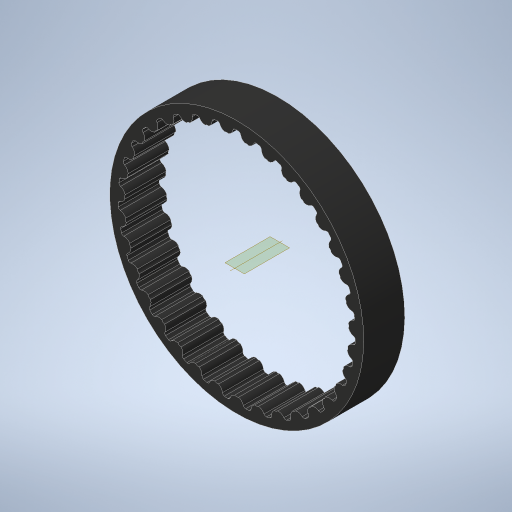
# Autodesk Inventor part: belt tooth
Saved by Autodesk Inventor 2023.3 (Build 273359000, 359)
## iProperties
Created: 2024-02-03
Part Number: belt tooth
Material: Rubber, Silicone
Document SubType Name: Modeling
Designer: mavericks
Density: 1.25 g/cm^3
Appearance: Rubber - Black
Author: mavericks
Autodesk Inventor part; units mm, degrees
(part 1 of 2)
ref_plane "YZ Plane" through (0, 0, 0) normal (1, 0, 0) x (0, 1, 0)
ref_plane "XZ Plane" through (0, 0, 0) normal (0, 1, 0) x (-1, 0, 0)
ref_plane "XY Plane" through (0, 0, 0) normal (0, 0, 1) x (1, 0, 0)
sketch "Sketch1" plane through (0, 0, 0) normal (0, 0, 1) x (1, 0, 0)
  line L0 (3.873, 1.9) -> (5, 1.9) construction
  arc A0 (3.3889, 2.275) -> (3.873, 1.9) centre (3.873, 2.4) ccw
  arc A1 (3.3889, 2.275) -> (2.3532, 3.341) centre (1.9365, 1.9) ccw
  arc A2 (1.5198, 3.341) -> (2.3532, 3.341) centre (1.9365, 4.0627) ccw
  arc A3 (1.5198, 3.341) -> (0.4841, 2.275) centre (1.9365, 1.9) ccw
  arc A4 (0, 1.9) -> (0.4841, 2.275) centre (0, 2.4) ccw
  line L1 (0, 0) -> (6.35, 0) construction
  line L2 (0, 1.9) -> (0, 0)
  line L3 (3.873, 1.9) -> (3.873, 0)
  line L4 (3.873, 0) -> (0, 0)
  dimension "d1" = 1.127
  dimension "d2" = 0.5
  dimension "d3" = 1.5
  dimension "d4" = 0.8333
  dimension "d5" = 1.5
  dimension "d6" = 0.5
  dimension "d7" = 1.9
  dimension "d8" = 2.4
  dimension "d9" = 1.9365
  dimension "d10" = 1.9365
  dimension "d11" = 1.6626
  dimension "d12" = 0.5
  dimension "d13" = 1.9
  dimension "d14" = 0
  dimension "d15" = 6.35
  dimension "d16" = 0.4841
  dimension "d17" = 1.0357
  dimension "d18" = 0.375
  dimension "d19" = 1.066
  constraints: 10 end point, 10 point on circle, 5 centre point, 2 perpendicular, 1 coincident, 1 horizontal, 1 point on line
  measures "d1" distance of L0.start L0.end
  measures "d2" radius of A0
  measures "d3" radius of A1
  measures "d4" radius of A2
  measures "d5" radius of A3
  measures "d6" radius of A4
  measures "d7" distance between parallel lines of L1 L0
  measures "d8" distance from line of L1 A4.centre
  measures "d9" horizontal distance of A2.centre A4.centre
  measures "d10" horizontal distance of A0.centre A2.centre
  measures "d11" vertical distance of A2.centre A0.centre
  measures "d12" vertical distance of A1.centre A0.centre
  measures "d13" distance from line of L1 A1.centre
  measures "d14" horizontal distance of L1.start A4.centre
  measures "d15" distance of L1.start L1.end
  measures "d16" horizontal distance of L0.start A0.start
  measures "d17" horizontal distance of A3.end A3.start
  measures "d18" vertical distance of L2.start A3.end
  measures "d19" vertical distance of A3.end A3.start
extrude "Extrusion1" add sketch "Sketch1" along normal mid plane 9
ref_plane "Work Plane1" through (0, 27.8521, 4.5) normal (0, -1, 0) x (1, 0, 0)
sketch "Sketch2" plane through (0, 27.8521, 4.5) normal (0, -1, 0) x (1, 0, 0)
  line L0 (1.5198, -9) -> (1.5198, 0) construction
  line L1 (2.3532, 0) -> (2.3532, 0) construction
  line L2 (2.3532, 0) -> (2.3532, -9) construction
  line L3 (1.5198, -9) -> (2.3532, -9) construction
  line L4 (3.873, -9) -> (0, -9) construction
  line L5 (1.9365, -9) -> (1.9365, 0)
  line L6 (2.3532, 0) -> (2.3532, 0) construction
  point P0 (0, -4.5)
  constraints: 2 end point, 1 midpoint, 1 point on line
pattern_circular "Circular Pattern1" count 35 over 360 about axis through (1.9365, 27.8521, -4.5) along (0, 0, 1) of "Extrusion1"
sketch "Sketch3" plane through (0, 0, 4.5) normal (0, 0, 1) x (1, 0, 0)
  arc A0 (3.3889, 2.275) -> (2.3532, 3.341) centre (1.9365, 1.9) ccw construction
  arc A1 (3.3889, 2.275) -> (3.873, 1.9) centre (3.873, 2.4) ccw construction
  line L0 (3.873, 1.9) -> (3.873, 0) construction
  line L1 (3.873, 0) -> (0, 0) construction
  line L2 (0, 0) -> (0, 1.9) construction
  arc A2 (0, 1.9) -> (0.4841, 2.275) centre (0, 2.4) ccw construction
  arc A3 (1.5198, 3.341) -> (0.4841, 2.275) centre (1.9365, 1.9) ccw construction
  arc A4 (1.5198, 3.341) -> (2.3532, 3.341) centre (1.9365, 4.0627) ccw construction
  arc A5 (7.9325, 2.9454) -> (6.7231, 3.8093) centre (6.5704, 2.3171) ccw construction
  arc A6 (7.9325, 2.9454) -> (8.4758, 2.6628) centre (8.3865, 3.1548) ccw construction
  line L3 (8.4758, 2.6628) -> (8.815, 0.7934) construction
  line L4 (8.815, 0.7934) -> (5.0043, 0.1018) construction
  line L5 (5.0043, 0.1018) -> (4.665, 1.9713) construction
  arc A7 (4.665, 1.9713) -> (5.0744, 2.4267) centre (4.5758, 2.4633) ccw construction
  arc A8 (5.9032, 3.6605) -> (5.0744, 2.4267) centre (6.5704, 2.3171) ccw construction
  arc A9 (5.9032, 3.6605) -> (6.7231, 3.8093) centre (6.1843, 4.445) ccw construction
  arc A10 (12.2834, 4.4163) -> (10.9392, 5.0503) centre (11.0554, 3.5548) ccw construction
  arc A11 (12.2834, 4.4163) -> (12.8684, 4.2353) centre (12.6927, 4.7034) ccw construction
  line L6 (12.8684, 4.2353) -> (13.536, 2.4564) construction
  line L7 (13.536, 2.4564) -> (9.91, 1.0956) construction
  line L8 (9.91, 1.0956) -> (9.2424, 2.8744) construction
  arc A12 (9.2424, 2.8744) -> (9.5639, 3.3956) centre (9.0667, 3.3425) ccw construction
  arc A13 (10.159, 4.7575) -> (9.5639, 3.3956) centre (11.0554, 3.5548) ccw construction
  arc A14 (10.159, 4.7575) -> (10.9392, 5.0503) centre (10.2955, 5.5796) ccw construction
  arc A15 (16.3018, 6.6404) -> (14.8659, 7.0243) centre (15.2473, 5.5736) ccw construction
  arc A16 (16.3018, 6.6404) -> (16.9097, 6.5668) centre (16.6532, 6.996) ccw construction
  line L9 (16.9097, 6.5668) -> (17.8842, 4.9357) construction
  line L10 (17.8842, 4.9357) -> (14.5594, 2.9493) construction
  line L11 (14.5594, 2.9493) -> (13.5849, 4.5803) construction
  arc A17 (13.5849, 4.5803) -> (13.8082, 5.1506) centre (13.3285, 5.0096) ccw construction
  arc A18 (14.1506, 6.5968) -> (13.8082, 5.1506) centre (15.2473, 5.5736) ccw construction
  arc A19 (14.1506, 6.5968) -> (14.8659, 7.0243) centre (14.1381, 7.4301) ccw construction
  arc A20 (19.8584, 9.5463) -> (18.3771, 9.6676) centre (19.0114, 8.3083) ccw construction
  arc A21 (19.8584, 9.5463) -> (20.4697, 9.5824) centre (20.1407, 9.9589) ccw construction
  line L12 (20.4697, 9.5824) -> (21.7198, 8.1516) construction
  line L13 (21.7198, 8.1516) -> (18.8032, 5.6034) construction
  line L14 (18.8032, 5.6034) -> (17.5531, 7.0342) construction
  arc A22 (17.5531, 7.0342) -> (17.6709, 7.6351) centre (17.2241, 7.4108) ccw construction
  arc A23 (17.7495, 9.1193) -> (17.6709, 7.6351) centre (19.0114, 8.3083) ccw construction
  arc A24 (17.7495, 9.1193) -> (18.3771, 9.6676) centre (17.5885, 9.937) ccw construction
  arc A25 (22.839, 13.0406) -> (21.3599, 12.8954) centre (22.2267, 11.6712) ccw construction
  arc A26 (22.839, 13.0406) -> (23.4341, 13.1852) centre (23.0431, 13.497) ccw construction
  line L15 (23.4341, 13.1852) -> (24.9195, 12.0006) construction
  line L16 (24.9195, 12.0006) -> (22.5048, 8.9726) construction
  line L17 (22.5048, 8.9726) -> (21.0193, 10.1572) construction
  arc A27 (21.0193, 10.1572) -> (21.0279, 10.7695) centre (20.6284, 10.469) ccw construction
  arc A28 (20.8403, 12.2439) -> (21.0279, 10.7695) centre (22.2267, 11.6712) ccw construction
  arc A29 (20.8403, 12.2439) -> (21.3599, 12.8954) centre (20.5358, 13.0196) ccw construction
  arc A30 (25.1478, 17.0109) -> (23.7183, 16.604) centre (24.7898, 15.5542) ccw construction
  arc A31 (25.1478, 17.0109) -> (25.7075, 17.2595) centre (25.2672, 17.4964) ccw construction
  line L18 (25.7075, 17.2595) -> (27.3806, 16.3591) construction
  line L19 (27.3806, 16.3591) -> (25.5453, 12.9486) construction
  line L20 (25.5453, 12.9486) -> (23.8722, 13.849) construction
  arc A32 (23.8722, 13.849) -> (23.7714, 14.453) centre (23.4319, 14.0859) ccw construction
  arc A33 (23.3235, 15.8701) -> (23.7714, 14.453) centre (24.7898, 15.5542) ccw construction
  arc A34 (23.3235, 15.8701) -> (23.7183, 16.604) centre (22.8854, 16.579) ccw construction
  arc A35 (26.7106, 21.3296) -> (25.3767, 20.674) centre (26.6184, 19.8325) ccw construction
  arc A36 (26.7106, 21.3296) -> (27.2168, 21.6742) centre (26.7413, 21.8287) ccw construction
  line L21 (27.2168, 21.6742) -> (29.0238, 21.0871) construction
  line L22 (29.0238, 21.0871) -> (27.827, 17.4036) construction
  line L23 (27.827, 17.4036) -> (26.02, 17.9908) construction
  arc A37 (26.02, 17.9908) -> (25.813, 18.5671) centre (25.5445, 18.1453) ccw construction
  arc A38 (25.1192, 19.8815) -> (25.813, 18.5671) centre (26.6184, 19.8325) ccw construction
  arc A39 (25.1192, 19.8815) -> (25.3767, 20.674) centre (24.5616, 20.5008) ccw construction
  arc A40 (27.4771, 25.858) -> (26.2817, 24.9748) centre (27.6537, 24.3685) ccw construction
  arc A41 (27.4771, 25.858) -> (27.9137, 26.2874) centre (27.4182, 26.3546) ccw construction
  line L24 (27.9137, 26.2874) -> (29.7965, 26.0324) construction
  line L25 (29.7965, 26.0324) -> (29.2766, 22.1945) construction
  line L26 (29.2766, 22.1945) -> (27.3938, 22.4495) construction
  arc A42 (27.3938, 22.4495) -> (27.0872, 22.9796) centre (26.8983, 22.5166) ccw construction
  arc A43 (26.1699, 24.149) -> (27.0872, 22.9796) centre (27.6537, 24.3685) ccw construction
  arc A44 (26.1699, 24.149) -> (26.2817, 24.9748) centre (25.5107, 24.6588) ccw construction
  arc A45 (27.4227, 30.4505) -> (26.4043, 29.3681) centre (27.8625, 29.0165) ccw construction
  arc A46 (27.4227, 30.4505) -> (27.7756, 30.951) centre (27.2761, 30.9286) ccw construction
  line L27 (27.7756, 30.951) -> (29.6737, 31.0362) construction
  line L28 (29.6737, 31.0362) -> (29.8474, 27.1672) construction
  line L29 (29.8474, 27.1672) -> (27.9494, 27.0819) construction
  arc A47 (27.9494, 27.0819) -> (27.553, 27.5487) centre (27.4499, 27.0595) ccw construction
  arc A48 (26.4417, 28.5356) -> (27.553, 27.5487) centre (27.8625, 29.0165) ccw construction
  arc A49 (26.4417, 28.5356) -> (26.4043, 29.3681) centre (25.702, 28.9194) ccw construction
  arc A50 (26.5492, 34.9595) -> (25.7404, 33.7126) centre (27.2379, 33.627) ccw construction
  arc A51 (26.5492, 34.9595) -> (26.807, 35.5149) centre (26.3196, 35.4037) ccw construction
  line L30 (26.807, 35.5149) -> (28.6594, 35.9377) construction
  line L31 (28.6594, 35.9377) -> (29.5212, 32.1619) construction
  line L32 (29.5212, 32.1619) -> (27.6688, 31.7391) construction
  arc A52 (27.6688, 31.7391) -> (27.1955, 32.1276) centre (27.1814, 31.6278) ccw construction
  arc A53 (25.9258, 32.9001) -> (27.1955, 32.1276) centre (27.2379, 33.627) ccw construction
  arc A54 (25.9258, 32.9001) -> (25.7404, 33.7126) centre (25.1295, 33.1458) ccw construction
  arc A55 (24.8845, 39.2401) -> (24.3114, 37.8687) centre (25.8002, 38.0519) ccw construction
  arc A56 (24.8845, 39.2401) -> (25.0391, 39.8326) centre (24.5793, 39.6361) ccw construction
  line L33 (25.0391, 39.8326) -> (26.7862, 40.5794) construction
  line L34 (26.7862, 40.5794) -> (28.3084, 37.018) construction
  line L35 (28.3084, 37.018) -> (26.5613, 36.2713) construction
  arc A57 (26.5613, 36.2713) -> (26.0262, 36.5691) centre (26.1015, 36.0748) ccw construction
  arc A58 (24.6389, 37.1025) -> (26.0262, 36.5691) centre (25.8002, 38.0519) ccw construction
  arc A59 (24.6389, 37.1025) -> (24.3114, 37.8687) centre (23.8116, 37.202) ccw construction
  arc A60 (22.4824, 43.1546) -> (22.1633, 41.703) centre (23.5954, 42.1491) ccw construction
  arc A61 (22.4824, 43.1546) -> (22.5286, 43.7652) centre (22.1113, 43.4898) ccw construction
  line L36 (22.5286, 43.7652) -> (24.1143, 44.8119) construction
  line L37 (24.1143, 44.8119) -> (26.2479, 41.5796) construction
  line L38 (26.2479, 41.5796) -> (24.6622, 40.5329) construction
  arc A62 (24.6622, 40.5329) -> (24.0826, 40.7304) centre (24.245, 40.2575) ccw construction
  arc A63 (22.6224, 41.0075) -> (24.0826, 40.7304) centre (23.5954, 42.1491) ccw construction
  arc A64 (22.6224, 41.0075) -> (22.1633, 41.703) centre (21.7905, 40.9577) ccw construction
  arc A65 (19.4198, 46.5773) -> (19.3651, 45.092) centre (20.6945, 45.7867) ccw construction
  arc A66 (19.4198, 46.5773) -> (19.3563, 47.1863) centre (18.9949, 46.8408) ccw construction
  line L39 (19.3563, 47.1863) -> (20.7296, 48.4994) construction
  line L40 (20.7296, 48.4994) -> (23.4061, 45.7) construction
  line L41 (23.4061, 45.7) -> (22.0328, 44.387) construction
  arc A67 (22.0328, 44.387) -> (21.4272, 44.4777) centre (21.6714, 44.0414) ccw construction
  arc A68 (19.941, 44.4897) -> (21.4272, 44.4777) centre (20.6945, 45.7867) ccw construction
  arc A69 (19.941, 44.4897) -> (19.3651, 45.092) centre (19.1314, 44.2921) ccw construction
  arc A70 (15.7954, 49.3981) -> (16.0067, 47.927) centre (17.1908, 48.8478) ccw construction
  arc A71 (15.7954, 49.3981) -> (15.6241, 49.9861) centre (15.3302, 49.5816) ccw construction
  line L42 (15.6241, 49.9861) -> (16.7409, 51.5232) construction
  line L43 (16.7409, 51.5232) -> (19.8742, 49.2467) construction
  line L44 (19.8742, 49.2467) -> (18.7574, 47.7096) construction
  arc A72 (18.7574, 47.7096) -> (18.1453, 47.6908) centre (18.4635, 47.3051) ccw construction
  arc A73 (16.6809, 47.4371) -> (18.1453, 47.6908) centre (17.1908, 48.8478) ccw construction
  arc A74 (16.6809, 47.4371) -> (16.0067, 47.927) centre (15.9196, 47.0982) ccw construction
  arc A75 (11.7254, 51.5265) -> (12.1961, 50.1167) centre (13.1967, 51.2342) ccw construction
  arc A76 (11.7254, 51.5265) -> (11.452, 52.0744) centre (11.235, 51.6239) ccw construction
  line L45 (11.452, 52.0744) -> (12.2764, 53.7862) construction
  line L46 (12.2764, 53.7862) -> (15.7658, 52.1058) construction
  line L47 (15.7658, 52.1058) -> (14.9414, 50.394) construction
  arc A77 (14.9414, 50.394) -> (14.3425, 50.2661) centre (14.7245, 49.9435) ccw construction
  arc A78 (12.9469, 49.7551) -> (14.3425, 50.2661) centre (13.1967, 51.2342) ccw construction
  arc A79 (12.9469, 49.7551) -> (12.1961, 50.1167) centre (12.2584, 49.2857) ccw construction
  arc A80 (7.3409, 52.8939) -> (8.0557, 51.5908) centre (8.8407, 52.869) ccw construction
  arc A81 (7.3409, 52.8939) -> (6.974, 53.3842) centre (6.841, 52.9022) ccw construction
  line L48 (6.974, 53.3842) -> (7.4795, 55.2157) construction
  line L49 (7.4795, 55.2157) -> (11.2129, 54.1853) construction
  line L50 (11.2129, 54.1853) -> (10.7074, 52.3538) construction
  arc A82 (10.7074, 52.3538) -> (10.141, 52.1211) centre (10.5744, 51.8718) ccw construction
  arc A83 (8.859, 51.3691) -> (10.141, 52.1211) centre (8.8407, 52.869) ccw construction
  arc A84 (8.859, 51.3691) -> (8.0557, 51.5908) centre (8.2654, 50.7843) ccw construction
  arc A85 (2.7827, 53.4565) -> (3.7187, 52.3019) centre (4.2628, 53.6998) ccw construction
  arc A86 (2.7827, 53.4565) -> (2.3341, 53.8733) centre (2.2893, 53.3754) ccw construction
  line L51 (2.3341, 53.8733) -> (2.5044, 55.7657) construction
  line L52 (2.5044, 55.7657) -> (6.3618, 55.4185) construction
  line L53 (6.3618, 55.4185) -> (6.1915, 53.5262) construction
  arc A87 (6.1915, 53.5262) -> (5.6757, 53.1961) centre (6.1467, 53.0282) ccw construction
  arc A88 (4.5486, 52.2272) -> (5.6757, 53.1961) centre (4.2628, 53.6998) ccw construction
  arc A89 (4.5486, 52.2272) -> (3.7187, 52.3019) centre (4.069, 51.5458) ccw construction
  arc A90 (-1.8027, 53.1961) -> (-0.6757, 52.2272) centre (-0.3898, 53.6998) ccw construction
  arc A91 (-1.8027, 53.1961) -> (-2.3185, 53.5262) centre (-2.2737, 53.0282) ccw construction
  line L54 (-2.3185, 53.5262) -> (-2.4888, 55.4185) construction
  line L55 (-2.4888, 55.4185) -> (1.3685, 55.7657) construction
  line L56 (1.3685, 55.7657) -> (1.5389, 53.8733) construction
  arc A92 (1.5389, 53.8733) -> (1.0903, 53.4565) centre (1.5837, 53.3754) ccw construction
  arc A93 (0.1543, 52.3019) -> (1.0903, 53.4565) centre (-0.3898, 53.6998) ccw construction
  arc A94 (0.1543, 52.3019) -> (-0.6757, 52.2272) centre (-0.196, 51.5458) ccw construction
  arc A95 (-6.268, 52.1211) -> (-4.986, 51.3691) centre (-4.9677, 52.869) ccw construction
  arc A96 (-6.268, 52.1211) -> (-6.8344, 52.3538) centre (-6.7014, 51.8718) ccw construction
  line L57 (-6.8344, 52.3538) -> (-7.3399, 54.1853) construction
  line L58 (-7.3399, 54.1853) -> (-3.6065, 55.2157) construction
  line L59 (-3.6065, 55.2157) -> (-3.101, 53.3842) construction
  arc A97 (-3.101, 53.3842) -> (-3.4679, 52.8939) centre (-2.968, 52.9022) ccw construction
  arc A98 (-4.1827, 51.5908) -> (-3.4679, 52.8939) centre (-4.9677, 52.869) ccw construction
  arc A99 (-4.1827, 51.5908) -> (-4.986, 51.3691) centre (-4.3924, 50.7843) ccw construction
  arc A100 (-10.4695, 50.2661) -> (-9.0739, 49.7551) centre (-9.3237, 51.2342) ccw construction
  arc A101 (-10.4695, 50.2661) -> (-11.0684, 50.394) centre (-10.8515, 49.9435) ccw construction
  line L60 (-11.0684, 50.394) -> (-11.8928, 52.1058) construction
  line L61 (-11.8928, 52.1058) -> (-8.4034, 53.7862) construction
  line L62 (-8.4034, 53.7862) -> (-7.579, 52.0744) construction
  arc A102 (-7.579, 52.0744) -> (-7.8525, 51.5265) centre (-7.3621, 51.6239) ccw construction
  arc A103 (-8.3231, 50.1167) -> (-7.8525, 51.5265) centre (-9.3237, 51.2342) ccw construction
  arc A104 (-8.3231, 50.1167) -> (-9.0739, 49.7551) centre (-8.3854, 49.2857) ccw construction
  arc A105 (-14.2724, 47.6908) -> (-12.8079, 47.4371) centre (-13.3178, 48.8478) ccw construction
  arc A106 (-14.2724, 47.6908) -> (-14.8844, 47.7096) centre (-14.5905, 47.3051) ccw construction
  line L63 (-14.8844, 47.7096) -> (-16.0012, 49.2467) construction
  line L64 (-16.0012, 49.2467) -> (-12.8679, 51.5232) construction
  line L65 (-12.8679, 51.5232) -> (-11.7511, 49.9861) construction
  arc A107 (-11.7511, 49.9861) -> (-11.9224, 49.3981) centre (-11.4572, 49.5816) ccw construction
  arc A108 (-12.1337, 47.927) -> (-11.9224, 49.3981) centre (-13.3178, 48.8478) ccw construction
  arc A109 (-12.1337, 47.927) -> (-12.8079, 47.4371) centre (-12.0466, 47.0982) ccw construction
  arc A110 (-17.5542, 44.4777) -> (-16.068, 44.4897) centre (-16.8216, 45.7867) ccw construction
  arc A111 (-17.5542, 44.4777) -> (-18.1598, 44.387) centre (-17.7984, 44.0414) ccw construction
  line L66 (-18.1598, 44.387) -> (-19.5331, 45.7) construction
  line L67 (-19.5331, 45.7) -> (-16.8566, 48.4994) construction
  line L68 (-16.8566, 48.4994) -> (-15.4833, 47.1863) construction
  arc A112 (-15.4833, 47.1863) -> (-15.5468, 46.5773) centre (-15.1219, 46.8408) ccw construction
  arc A113 (-15.4921, 45.092) -> (-15.5468, 46.5773) centre (-16.8216, 45.7867) ccw construction
  arc A114 (-15.4921, 45.092) -> (-16.068, 44.4897) centre (-15.2584, 44.2921) ccw construction
  arc A115 (-20.2096, 40.7304) -> (-18.7494, 41.0075) centre (-19.7225, 42.1491) ccw construction
  arc A116 (-20.2096, 40.7304) -> (-20.7893, 40.5329) centre (-20.372, 40.2575) ccw construction
  line L69 (-20.7893, 40.5329) -> (-22.3749, 41.5796) construction
  line L70 (-22.3749, 41.5796) -> (-20.2413, 44.8119) construction
  line L71 (-20.2413, 44.8119) -> (-18.6556, 43.7652) construction
  arc A117 (-18.6556, 43.7652) -> (-18.6094, 43.1546) centre (-18.2384, 43.4898) ccw construction
  arc A118 (-18.2903, 41.703) -> (-18.6094, 43.1546) centre (-19.7225, 42.1491) ccw construction
  arc A119 (-18.2903, 41.703) -> (-18.7494, 41.0075) centre (-17.9176, 40.9577) ccw construction
  arc A120 (-22.1532, 36.5691) -> (-20.766, 37.1025) centre (-21.9272, 38.0519) ccw construction
  arc A121 (-22.1532, 36.5691) -> (-22.6883, 36.2713) centre (-22.2285, 36.0748) ccw construction
  line L72 (-22.6883, 36.2713) -> (-24.4354, 37.018) construction
  line L73 (-24.4354, 37.018) -> (-22.9132, 40.5794) construction
  line L74 (-22.9132, 40.5794) -> (-21.1661, 39.8326) construction
  arc A122 (-21.1661, 39.8326) -> (-21.0116, 39.2401) centre (-20.7063, 39.6361) ccw construction
  arc A123 (-20.4384, 37.8687) -> (-21.0116, 39.2401) centre (-21.9272, 38.0519) ccw construction
  arc A124 (-20.4384, 37.8687) -> (-20.766, 37.1025) centre (-19.9386, 37.202) ccw construction
  arc A125 (-23.3225, 32.1276) -> (-22.0528, 32.9001) centre (-23.365, 33.627) ccw construction
  arc A126 (-23.3225, 32.1276) -> (-23.7959, 31.7391) centre (-23.3084, 31.6278) ccw construction
  line L75 (-23.7959, 31.7391) -> (-25.6482, 32.1619) construction
  line L76 (-25.6482, 32.1619) -> (-24.7864, 35.9377) construction
  line L77 (-24.7864, 35.9377) -> (-22.934, 35.5149) construction
  arc A127 (-22.934, 35.5149) -> (-22.6762, 34.9595) centre (-22.4466, 35.4037) ccw construction
  arc A128 (-21.8674, 33.7126) -> (-22.6762, 34.9595) centre (-23.365, 33.627) ccw construction
  arc A129 (-21.8674, 33.7126) -> (-22.0528, 32.9001) centre (-21.2565, 33.1458) ccw construction
  arc A130 (-23.68, 27.5487) -> (-22.5687, 28.5356) centre (-23.9895, 29.0165) ccw construction
  arc A131 (-23.68, 27.5487) -> (-24.0764, 27.0819) centre (-23.5769, 27.0595) ccw construction
  line L78 (-24.0764, 27.0819) -> (-25.9745, 27.1672) construction
  line L79 (-25.9745, 27.1672) -> (-25.8007, 31.0362) construction
  line L80 (-25.8007, 31.0362) -> (-23.9026, 30.951) construction
  arc A132 (-23.9026, 30.951) -> (-23.5497, 30.4505) centre (-23.4031, 30.9286) ccw construction
  arc A133 (-22.5313, 29.3681) -> (-23.5497, 30.4505) centre (-23.9895, 29.0165) ccw construction
  arc A134 (-22.5313, 29.3681) -> (-22.5687, 28.5356) centre (-21.829, 28.9194) ccw construction
  arc A135 (-23.2142, 22.9796) -> (-22.2969, 24.149) centre (-23.7808, 24.3685) ccw construction
  arc A136 (-23.2142, 22.9796) -> (-23.5208, 22.4495) centre (-23.0253, 22.5166) ccw construction
  line L81 (-23.5208, 22.4495) -> (-25.4036, 22.1945) construction
  line L82 (-25.4036, 22.1945) -> (-25.9235, 26.0324) construction
  line L83 (-25.9235, 26.0324) -> (-24.0407, 26.2874) construction
  arc A137 (-24.0407, 26.2874) -> (-23.6041, 25.858) centre (-23.5452, 26.3546) ccw construction
  arc A138 (-22.4088, 24.9748) -> (-23.6041, 25.858) centre (-23.7808, 24.3685) ccw construction
  arc A139 (-22.4088, 24.9748) -> (-22.2969, 24.149) centre (-21.6377, 24.6588) ccw construction
  arc A140 (-21.94, 18.5671) -> (-21.2462, 19.8815) centre (-22.7454, 19.8325) ccw construction
  arc A141 (-21.94, 18.5671) -> (-22.147, 17.9908) centre (-21.6715, 18.1453) ccw construction
  line L84 (-22.147, 17.9908) -> (-23.954, 17.4036) construction
  line L85 (-23.954, 17.4036) -> (-25.1509, 21.0871) construction
  line L86 (-25.1509, 21.0871) -> (-23.3438, 21.6742) construction
  arc A142 (-23.3438, 21.6742) -> (-22.8376, 21.3296) centre (-22.8683, 21.8287) ccw construction
  arc A143 (-21.5038, 20.674) -> (-22.8376, 21.3296) centre (-22.7454, 19.8325) ccw construction
  arc A144 (-21.5038, 20.674) -> (-21.2462, 19.8815) centre (-20.6886, 20.5008) ccw construction
  arc A145 (-19.8984, 14.453) -> (-19.4505, 15.8701) centre (-20.9168, 15.5542) ccw construction
  arc A146 (-19.8984, 14.453) -> (-19.9992, 13.849) centre (-19.5589, 14.0859) ccw construction
  line L87 (-19.9992, 13.849) -> (-21.6723, 12.9486) construction
  line L88 (-21.6723, 12.9486) -> (-23.5076, 16.3591) construction
  line L89 (-23.5076, 16.3591) -> (-21.8345, 17.2595) construction
  arc A147 (-21.8345, 17.2595) -> (-21.2748, 17.0109) centre (-21.3942, 17.4964) ccw construction
  arc A148 (-19.8454, 16.604) -> (-21.2748, 17.0109) centre (-20.9168, 15.5542) ccw construction
  arc A149 (-19.8454, 16.604) -> (-19.4505, 15.8701) centre (-19.0124, 16.579) ccw construction
  arc A150 (-17.155, 10.7695) -> (-16.9673, 12.2439) centre (-18.3537, 11.6712) ccw construction
  arc A151 (-17.155, 10.7695) -> (-17.1463, 10.1572) centre (-16.7554, 10.469) ccw construction
  line L90 (-17.1463, 10.1572) -> (-18.6318, 8.9726) construction
  line L91 (-18.6318, 8.9726) -> (-21.0466, 12.0006) construction
  line L92 (-21.0466, 12.0006) -> (-19.5611, 13.1852) construction
  arc A152 (-19.5611, 13.1852) -> (-18.966, 13.0406) centre (-19.1702, 13.497) ccw construction
  arc A153 (-17.4869, 12.8954) -> (-18.966, 13.0406) centre (-18.3537, 11.6712) ccw construction
  arc A154 (-17.4869, 12.8954) -> (-16.9673, 12.2439) centre (-16.6629, 13.0196) ccw construction
  arc A155 (-13.7979, 7.6351) -> (-13.8766, 9.1193) centre (-15.1384, 8.3083) ccw construction
  arc A156 (-13.7979, 7.6351) -> (-13.6801, 7.0342) centre (-13.3511, 7.4108) ccw construction
  line L93 (-13.6801, 7.0342) -> (-14.9302, 5.6034) construction
  line L94 (-14.9302, 5.6034) -> (-17.8468, 8.1516) construction
  line L95 (-17.8468, 8.1516) -> (-16.5967, 9.5824) construction
  arc A157 (-16.5967, 9.5824) -> (-15.9854, 9.5463) centre (-16.2678, 9.9589) ccw construction
  arc A158 (-14.5041, 9.6676) -> (-15.9854, 9.5463) centre (-15.1384, 8.3083) ccw construction
  arc A159 (-14.5041, 9.6676) -> (-13.8766, 9.1193) centre (-13.7155, 9.937) ccw construction
  arc A160 (-9.9352, 5.1506) -> (-10.2776, 6.5968) centre (-11.3743, 5.5736) ccw construction
  arc A161 (-9.9352, 5.1506) -> (-9.712, 4.5803) centre (-9.4555, 5.0096) ccw construction
  line L96 (-9.712, 4.5803) -> (-10.6865, 2.9493) construction
  line L97 (-10.6865, 2.9493) -> (-14.0112, 4.9357) construction
  line L98 (-14.0112, 4.9357) -> (-13.0367, 6.5668) construction
  arc A162 (-13.0367, 6.5668) -> (-12.4288, 6.6404) centre (-12.7803, 6.996) ccw construction
  arc A163 (-10.9929, 7.0243) -> (-12.4288, 6.6404) centre (-11.3743, 5.5736) ccw construction
  arc A164 (-10.9929, 7.0243) -> (-10.2776, 6.5968) centre (-10.2651, 7.4301) ccw construction
  arc A165 (-5.6909, 3.3956) -> (-6.286, 4.7575) centre (-7.1824, 3.5548) ccw construction
  arc A166 (-5.6909, 3.3956) -> (-5.3694, 2.8744) centre (-5.1937, 3.3425) ccw construction
  line L99 (-5.3694, 2.8744) -> (-6.037, 1.0956) construction
  line L100 (-6.037, 1.0956) -> (-9.6631, 2.4564) construction
  line L101 (-9.6631, 2.4564) -> (-8.9954, 4.2353) construction
  arc A167 (-8.9954, 4.2353) -> (-8.4104, 4.4163) centre (-8.8198, 4.7034) ccw construction
  arc A168 (-7.0662, 5.0503) -> (-8.4104, 4.4163) centre (-7.1824, 3.5548) ccw construction
  arc A169 (-7.0662, 5.0503) -> (-6.286, 4.7575) centre (-6.4225, 5.5796) ccw construction
  arc A170 (-1.2015, 2.4267) -> (-2.0302, 3.6605) centre (-2.6974, 2.3171) ccw construction
  arc A171 (-1.2015, 2.4267) -> (-0.7921, 1.9713) centre (-0.7028, 2.4633) ccw construction
  line L102 (-0.7921, 1.9713) -> (-1.1313, 0.1018) construction
  line L103 (-1.1313, 0.1018) -> (-4.9421, 0.7934) construction
  line L104 (-4.9421, 0.7934) -> (-4.6028, 2.6628) construction
  arc A172 (-4.6028, 2.6628) -> (-4.0595, 2.9454) centre (-4.5135, 3.1548) ccw construction
  arc A173 (-2.8501, 3.8093) -> (-4.0595, 2.9454) centre (-2.6974, 2.3171) ccw construction
  arc A174 (-2.8501, 3.8093) -> (-2.0302, 3.6605) centre (-2.3113, 4.445) ccw construction
  arc A175 (3.3889, 2.275) -> (2.3532, 3.341) centre (1.9365, 1.9) ccw construction
  arc A176 (3.3889, 2.275) -> (3.873, 1.9) centre (3.873, 2.4) ccw construction
  line L105 (3.873, 1.9) -> (3.873, 0) construction
  line L106 (3.873, 0) -> (0, 0) construction
  line L107 (0, 0) -> (0, 1.9) construction
  arc A177 (0, 1.9) -> (0.4841, 2.275) centre (0, 2.4) ccw construction
  arc A178 (1.5198, 3.341) -> (0.4841, 2.275) centre (1.9365, 1.9) ccw construction
  arc A179 (1.5198, 3.341) -> (2.3532, 3.341) centre (1.9365, 4.0627) ccw construction
  arc A180 (7.9325, 2.9454) -> (6.7231, 3.8093) centre (6.5704, 2.3171) ccw construction
  arc A181 (7.9325, 2.9454) -> (8.4758, 2.6628) centre (8.3865, 3.1548) ccw construction
  line L108 (8.4758, 2.6628) -> (8.815, 0.7934) construction
  line L109 (8.815, 0.7934) -> (5.0043, 0.1018) construction
  line L110 (5.0043, 0.1018) -> (4.665, 1.9713) construction
  arc A182 (4.665, 1.9713) -> (5.0744, 2.4267) centre (4.5758, 2.4633) ccw construction
  arc A183 (5.9032, 3.6605) -> (5.0744, 2.4267) centre (6.5704, 2.3171) ccw construction
  arc A184 (5.9032, 3.6605) -> (6.7231, 3.8093) centre (6.1843, 4.445) ccw construction
  arc A185 (12.2834, 4.4163) -> (10.9392, 5.0503) centre (11.0554, 3.5548) ccw construction
  arc A186 (12.2834, 4.4163) -> (12.8684, 4.2353) centre (12.6927, 4.7034) ccw construction
  line L111 (12.8684, 4.2353) -> (13.536, 2.4564) construction
  line L112 (13.536, 2.4564) -> (9.91, 1.0956) construction
  line L113 (9.91, 1.0956) -> (9.2424, 2.8744) construction
  arc A187 (9.2424, 2.8744) -> (9.5639, 3.3956) centre (9.0667, 3.3425) ccw construction
  arc A188 (10.159, 4.7575) -> (9.5639, 3.3956) centre (11.0554, 3.5548) ccw construction
  arc A189 (10.159, 4.7575) -> (10.9392, 5.0503) centre (10.2955, 5.5796) ccw construction
  arc A190 (16.3018, 6.6404) -> (14.8659, 7.0243) centre (15.2473, 5.5736) ccw construction
  arc A191 (16.3018, 6.6404) -> (16.9097, 6.5668) centre (16.6532, 6.996) ccw construction
  line L114 (16.9097, 6.5668) -> (17.8842, 4.9357) construction
  line L115 (17.8842, 4.9357) -> (14.5594, 2.9493) construction
  line L116 (14.5594, 2.9493) -> (13.5849, 4.5803) construction
  arc A192 (13.5849, 4.5803) -> (13.8082, 5.1506) centre (13.3285, 5.0096) ccw construction
  arc A193 (14.1506, 6.5968) -> (13.8082, 5.1506) centre (15.2473, 5.5736) ccw construction
  arc A194 (14.1506, 6.5968) -> (14.8659, 7.0243) centre (14.1381, 7.4301) ccw construction
  arc A195 (19.8584, 9.5463) -> (18.3771, 9.6676) centre (19.0114, 8.3083) ccw construction
  arc A196 (19.8584, 9.5463) -> (20.4697, 9.5824) centre (20.1407, 9.9589) ccw construction
  line L117 (20.4697, 9.5824) -> (21.7198, 8.1516) construction
  line L118 (21.7198, 8.1516) -> (18.8032, 5.6034) construction
  line L119 (18.8032, 5.6034) -> (17.5531, 7.0342) construction
  arc A197 (17.5531, 7.0342) -> (17.6709, 7.6351) centre (17.2241, 7.4108) ccw construction
  arc A198 (17.7495, 9.1193) -> (17.6709, 7.6351) centre (19.0114, 8.3083) ccw construction
  arc A199 (17.7495, 9.1193) -> (18.3771, 9.6676) centre (17.5885, 9.937) ccw construction
  arc A200 (22.839, 13.0406) -> (21.3599, 12.8954) centre (22.2267, 11.6712) ccw construction
  arc A201 (22.839, 13.0406) -> (23.4341, 13.1852) centre (23.0431, 13.497) ccw construction
  line L120 (23.4341, 13.1852) -> (24.9195, 12.0006) construction
  line L121 (24.9195, 12.0006) -> (22.5048, 8.9726) construction
  line L122 (22.5048, 8.9726) -> (21.0193, 10.1572) construction
  arc A202 (21.0193, 10.1572) -> (21.0279, 10.7695) centre (20.6284, 10.469) ccw construction
  arc A203 (20.8403, 12.2439) -> (21.0279, 10.7695) centre (22.2267, 11.6712) ccw construction
  arc A204 (20.8403, 12.2439) -> (21.3599, 12.8954) centre (20.5358, 13.0196) ccw construction
  arc A205 (25.1478, 17.0109) -> (23.7183, 16.604) centre (24.7898, 15.5542) ccw construction
  arc A206 (25.1478, 17.0109) -> (25.7075, 17.2595) centre (25.2672, 17.4964) ccw construction
  line L123 (25.7075, 17.2595) -> (27.3806, 16.3591) construction
  line L124 (27.3806, 16.3591) -> (25.5453, 12.9486) construction
  line L125 (25.5453, 12.9486) -> (23.8722, 13.849) construction
  arc A207 (23.8722, 13.849) -> (23.7714, 14.453) centre (23.4319, 14.0859) ccw construction
  arc A208 (23.3235, 15.8701) -> (23.7714, 14.453) centre (24.7898, 15.5542) ccw construction
  arc A209 (23.3235, 15.8701) -> (23.7183, 16.604) centre (22.8854, 16.579) ccw construction
  arc A210 (26.7106, 21.3296) -> (25.3767, 20.674) centre (26.6184, 19.8325) ccw construction
  arc A211 (26.7106, 21.3296) -> (27.2168, 21.6742) centre (26.7413, 21.8287) ccw construction
  line L126 (27.2168, 21.6742) -> (29.0238, 21.0871) construction
  line L127 (29.0238, 21.0871) -> (27.827, 17.4036) construction
  line L128 (27.827, 17.4036) -> (26.02, 17.9908) construction
  arc A212 (26.02, 17.9908) -> (25.813, 18.5671) centre (25.5445, 18.1453) ccw construction
  arc A213 (25.1192, 19.8815) -> (25.813, 18.5671) centre (26.6184, 19.8325) ccw construction
  arc A214 (25.1192, 19.8815) -> (25.3767, 20.674) centre (24.5616, 20.5008) ccw construction
  arc A215 (27.4771, 25.858) -> (26.2817, 24.9748) centre (27.6537, 24.3685) ccw construction
  arc A216 (27.4771, 25.858) -> (27.9137, 26.2874) centre (27.4182, 26.3546) ccw construction
  line L129 (27.9137, 26.2874) -> (29.7965, 26.0324) construction
  line L130 (29.7965, 26.0324) -> (29.2766, 22.1945) construction
  line L131 (29.2766, 22.1945) -> (27.3938, 22.4495) construction
  arc A217 (27.3938, 22.4495) -> (27.0872, 22.9796) centre (26.8983, 22.5166) ccw construction
  arc A218 (26.1699, 24.149) -> (27.0872, 22.9796) centre (27.6537, 24.3685) ccw construction
  arc A219 (26.1699, 24.149) -> (26.2817, 24.9748) centre (25.5107, 24.6588) ccw construction
  arc A220 (27.4227, 30.4505) -> (26.4043, 29.3681) centre (27.8625, 29.0165) ccw construction
  arc A221 (27.4227, 30.4505) -> (27.7756, 30.951) centre (27.2761, 30.9286) ccw construction
  line L132 (27.7756, 30.951) -> (29.6737, 31.0362) construction
  line L133 (29.6737, 31.0362) -> (29.8474, 27.1672) construction
  line L134 (29.8474, 27.1672) -> (27.9494, 27.0819) construction
  arc A222 (27.9494, 27.0819) -> (27.553, 27.5487) centre (27.4499, 27.0595) ccw construction
  arc A223 (26.4417, 28.5356) -> (27.553, 27.5487) centre (27.8625, 29.0165) ccw construction
  arc A224 (26.4417, 28.5356) -> (26.4043, 29.3681) centre (25.702, 28.9194) ccw construction
  arc A225 (26.5492, 34.9595) -> (25.7404, 33.7126) centre (27.2379, 33.627) ccw construction
  arc A226 (26.5492, 34.9595) -> (26.807, 35.5149) centre (26.3196, 35.4037) ccw construction
  line L135 (26.807, 35.5149) -> (28.6594, 35.9377) construction
  line L136 (28.6594, 35.9377) -> (29.5212, 32.1619) construction
  line L137 (29.5212, 32.1619) -> (27.6688, 31.7391) construction
  arc A227 (27.6688, 31.7391) -> (27.1955, 32.1276) centre (27.1814, 31.6278) ccw construction
  arc A228 (25.9258, 32.9001) -> (27.1955, 32.1276) centre (27.2379, 33.627) ccw construction
  arc A229 (25.9258, 32.9001) -> (25.7404, 33.7126) centre (25.1295, 33.1458) ccw construction
  arc A230 (24.8845, 39.2401) -> (24.3114, 37.8687) centre (25.8002, 38.0519) ccw construction
  arc A231 (24.8845, 39.2401) -> (25.0391, 39.8326) centre (24.5793, 39.6361) ccw construction
  line L138 (25.0391, 39.8326) -> (26.7862, 40.5794) construction
  line L139 (26.7862, 40.5794) -> (28.3084, 37.018) construction
  line L140 (28.3084, 37.018) -> (26.5613, 36.2713) construction
  arc A232 (26.5613, 36.2713) -> (26.0262, 36.5691) centre (26.1015, 36.0748) ccw construction
  arc A233 (24.6389, 37.1025) -> (26.0262, 36.5691) centre (25.8002, 38.0519) ccw construction
  arc A234 (24.6389, 37.1025) -> (24.3114, 37.8687) centre (23.8116, 37.202) ccw construction
  arc A235 (22.4824, 43.1546) -> (22.1633, 41.703) centre (23.5954, 42.1491) ccw construction
  arc A236 (22.4824, 43.1546) -> (22.5286, 43.7652) centre (22.1113, 43.4898) ccw construction
  line L141 (22.5286, 43.7652) -> (24.1143, 44.8119) construction
  line L142 (24.1143, 44.8119) -> (26.2479, 41.5796) construction
  line L143 (26.2479, 41.5796) -> (24.6622, 40.5329) construction
  arc A237 (24.6622, 40.5329) -> (24.0826, 40.7304) centre (24.245, 40.2575) ccw construction
  arc A238 (22.6224, 41.0075) -> (24.0826, 40.7304) centre (23.5954, 42.1491) ccw construction
  arc A239 (22.6224, 41.0075) -> (22.1633, 41.703) centre (21.7905, 40.9577) ccw construction
  arc A240 (19.4198, 46.5773) -> (19.3651, 45.092) centre (20.6945, 45.7867) ccw construction
  arc A241 (19.4198, 46.5773) -> (19.3563, 47.1863) centre (18.9949, 46.8408) ccw construction
  line L144 (19.3563, 47.1863) -> (20.7296, 48.4994) construction
  line L145 (20.7296, 48.4994) -> (23.4061, 45.7) construction
  line L146 (23.4061, 45.7) -> (22.0328, 44.387) construction
  arc A242 (22.0328, 44.387) -> (21.4272, 44.4777) centre (21.6714, 44.0414) ccw construction
  arc A243 (19.941, 44.4897) -> (21.4272, 44.4777) centre (20.6945, 45.7867) ccw construction
  arc A244 (19.941, 44.4897) -> (19.3651, 45.092) centre (19.1314, 44.2921) ccw construction
  arc A245 (15.7954, 49.3981) -> (16.0067, 47.927) centre (17.1908, 48.8478) ccw construction
  arc A246 (15.7954, 49.3981) -> (15.6241, 49.9861) centre (15.3302, 49.5816) ccw construction
  line L147 (15.6241, 49.9861) -> (16.7409, 51.5232) construction
  line L148 (16.7409, 51.5232) -> (19.8742, 49.2467) construction
  line L149 (19.8742, 49.2467) -> (18.7574, 47.7096) construction
  arc A247 (18.7574, 47.7096) -> (18.1453, 47.6908) centre (18.4635, 47.3051) ccw construction
  arc A248 (16.6809, 47.4371) -> (18.1453, 47.6908) centre (17.1908, 48.8478) ccw construction
  arc A249 (16.6809, 47.4371) -> (16.0067, 47.927) centre (15.9196, 47.0982) ccw construction
  arc A250 (11.7254, 51.5265) -> (12.1961, 50.1167) centre (13.1967, 51.2342) ccw construction
  arc A251 (11.7254, 51.5265) -> (11.452, 52.0744) centre (11.235, 51.6239) ccw construction
  line L150 (11.452, 52.0744) -> (12.2764, 53.7862) construction
  line L151 (12.2764, 53.7862) -> (15.7658, 52.1058) construction
  line L152 (15.7658, 52.1058) -> (14.9414, 50.394) construction
  arc A252 (14.9414, 50.394) -> (14.3425, 50.2661) centre (14.7245, 49.9435) ccw construction
  arc A253 (12.9469, 49.7551) -> (14.3425, 50.2661) centre (13.1967, 51.2342) ccw construction
  arc A254 (12.9469, 49.7551) -> (12.1961, 50.1167) centre (12.2584, 49.2857) ccw construction
  arc A255 (7.3409, 52.8939) -> (8.0557, 51.5908) centre (8.8407, 52.869) ccw construction
  arc A256 (7.3409, 52.8939) -> (6.974, 53.3842) centre (6.841, 52.9022) ccw construction
  line L153 (6.974, 53.3842) -> (7.4795, 55.2157) construction
  line L154 (7.4795, 55.2157) -> (11.2129, 54.1853) construction
  line L155 (11.2129, 54.1853) -> (10.7074, 52.3538) construction
  arc A257 (10.7074, 52.3538) -> (10.141, 52.1211) centre (10.5744, 51.8718) ccw construction
  arc A258 (8.859, 51.3691) -> (10.141, 52.1211) centre (8.8407, 52.869) ccw construction
  arc A259 (8.859, 51.3691) -> (8.0557, 51.5908) centre (8.2654, 50.7843) ccw construction
  arc A260 (2.7827, 53.4565) -> (3.7187, 52.3019) centre (4.2628, 53.6998) ccw construction
  arc A261 (2.7827, 53.4565) -> (2.3341, 53.8733) centre (2.2893, 53.3754) ccw construction
  line L156 (2.3341, 53.8733) -> (2.5044, 55.7657) construction
  line L157 (2.5044, 55.7657) -> (6.3618, 55.4185) construction
  line L158 (6.3618, 55.4185) -> (6.1915, 53.5262) construction
  arc A262 (6.1915, 53.5262) -> (5.6757, 53.1961) centre (6.1467, 53.0282) ccw construction
  arc A263 (4.5486, 52.2272) -> (5.6757, 53.1961) centre (4.2628, 53.6998) ccw construction
  arc A264 (4.5486, 52.2272) -> (3.7187, 52.3019) centre (4.069, 51.5458) ccw construction
  arc A265 (-1.8027, 53.1961) -> (-0.6757, 52.2272) centre (-0.3898, 53.6998) ccw construction
  arc A266 (-1.8027, 53.1961) -> (-2.3185, 53.5262) centre (-2.2737, 53.0282) ccw construction
  line L159 (-2.3185, 53.5262) -> (-2.4888, 55.4185) construction
  line L160 (-2.4888, 55.4185) -> (1.3685, 55.7657) construction
  line L161 (1.3685, 55.7657) -> (1.5389, 53.8733) construction
  arc A267 (1.5389, 53.8733) -> (1.0903, 53.4565) centre (1.5837, 53.3754) ccw construction
  arc A268 (0.1543, 52.3019) -> (1.0903, 53.4565) centre (-0.3898, 53.6998) ccw construction
  arc A269 (0.1543, 52.3019) -> (-0.6757, 52.2272) centre (-0.196, 51.5458) ccw construction
  arc A270 (-6.268, 52.1211) -> (-4.986, 51.3691) centre (-4.9677, 52.869) ccw construction
  arc A271 (-6.268, 52.1211) -> (-6.8344, 52.3538) centre (-6.7014, 51.8718) ccw construction
  line L162 (-6.8344, 52.3538) -> (-7.3399, 54.1853) construction
  line L163 (-7.3399, 54.1853) -> (-3.6065, 55.2157) construction
  line L164 (-3.6065, 55.2157) -> (-3.101, 53.3842) construction
  arc A272 (-3.101, 53.3842) -> (-3.4679, 52.8939) centre (-2.968, 52.9022) ccw construction
  arc A273 (-4.1827, 51.5908) -> (-3.4679, 52.8939) centre (-4.9677, 52.869) ccw construction
  arc A274 (-4.1827, 51.5908) -> (-4.986, 51.3691) centre (-4.3924, 50.7843) ccw construction
  arc A275 (-10.4695, 50.2661) -> (-9.0739, 49.7551) centre (-9.3237, 51.2342) ccw construction
  arc A276 (-10.4695, 50.2661) -> (-11.0684, 50.394) centre (-10.8515, 49.9435) ccw construction
  line L165 (-11.0684, 50.394) -> (-11.8928, 52.1058) construction
  line L166 (-11.8928, 52.1058) -> (-8.4034, 53.7862) construction
  line L167 (-8.4034, 53.7862) -> (-7.579, 52.0744) construction
  arc A277 (-7.579, 52.0744) -> (-7.8525, 51.5265) centre (-7.3621, 51.6239) ccw construction
  arc A278 (-8.3231, 50.1167) -> (-7.8525, 51.5265) centre (-9.3237, 51.2342) ccw construction
  arc A279 (-8.3231, 50.1167) -> (-9.0739, 49.7551) centre (-8.3854, 49.2857) ccw construction
  arc A280 (-14.2724, 47.6908) -> (-12.8079, 47.4371) centre (-13.3178, 48.8478) ccw construction
  arc A281 (-14.2724, 47.6908) -> (-14.8844, 47.7096) centre (-14.5905, 47.3051) ccw construction
  line L168 (-14.8844, 47.7096) -> (-16.0012, 49.2467) construction
  line L169 (-16.0012, 49.2467) -> (-12.8679, 51.5232) construction
  line L170 (-12.8679, 51.5232) -> (-11.7511, 49.9861) construction
  arc A282 (-11.7511, 49.9861) -> (-11.9224, 49.3981) centre (-11.4572, 49.5816) ccw construction
  arc A283 (-12.1337, 47.927) -> (-11.9224, 49.3981) centre (-13.3178, 48.8478) ccw construction
  arc A284 (-12.1337, 47.927) -> (-12.8079, 47.4371) centre (-12.0466, 47.0982) ccw construction
  arc A285 (-17.5542, 44.4777) -> (-16.068, 44.4897) centre (-16.8216, 45.7867) ccw construction
  arc A286 (-17.5542, 44.4777) -> (-18.1598, 44.387) centre (-17.7984, 44.0414) ccw construction
  line L171 (-18.1598, 44.387) -> (-19.5331, 45.7) construction
  line L172 (-19.5331, 45.7) -> (-16.8566, 48.4994) construction
  line L173 (-16.8566, 48.4994) -> (-15.4833, 47.1863) construction
  arc A287 (-15.4833, 47.1863) -> (-15.5468, 46.5773) centre (-15.1219, 46.8408) ccw construction
  arc A288 (-15.4921, 45.092) -> (-15.5468, 46.5773) centre (-16.8216, 45.7867) ccw construction
  arc A289 (-15.4921, 45.092) -> (-16.068, 44.4897) centre (-15.2584, 44.2921) ccw construction
  arc A290 (-20.2096, 40.7304) -> (-18.7494, 41.0075) centre (-19.7225, 42.1491) ccw construction
  arc A291 (-20.2096, 40.7304) -> (-20.7893, 40.5329) centre (-20.372, 40.2575) ccw construction
  line L174 (-20.7893, 40.5329) -> (-22.3749, 41.5796) construction
  line L175 (-22.3749, 41.5796) -> (-20.2413, 44.8119) construction
  line L176 (-20.2413, 44.8119) -> (-18.6556, 43.7652) construction
  arc A292 (-18.6556, 43.7652) -> (-18.6094, 43.1546) centre (-18.2384, 43.4898) ccw construction
  arc A293 (-18.2903, 41.703) -> (-18.6094, 43.1546) centre (-19.7225, 42.1491) ccw construction
  arc A294 (-18.2903, 41.703) -> (-18.7494, 41.0075) centre (-17.9176, 40.9577) ccw construction
  arc A295 (-22.1532, 36.5691) -> (-20.766, 37.1025) centre (-21.9272, 38.0519) ccw construction
  arc A296 (-22.1532, 36.5691) -> (-22.6883, 36.2713) centre (-22.2285, 36.0748) ccw construction
  line L177 (-22.6883, 36.2713) -> (-24.4354, 37.018) construction
  line L178 (-24.4354, 37.018) -> (-22.9132, 40.5794) construction
  line L179 (-22.9132, 40.5794) -> (-21.1661, 39.8326) construction
  arc A297 (-21.1661, 39.8326) -> (-21.0116, 39.2401) centre (-20.7063, 39.6361) ccw construction
  arc A298 (-20.4384, 37.8687) -> (-21.0116, 39.2401) centre (-21.9272, 38.0519) ccw construction
  arc A299 (-20.4384, 37.8687) -> (-20.766, 37.1025) centre (-19.9386, 37.202) ccw construction
  arc A300 (-23.3225, 32.1276) -> (-22.0528, 32.9001) centre (-23.365, 33.627) ccw construction
  arc A301 (-23.3225, 32.1276) -> (-23.7959, 31.7391) centre (-23.3084, 31.6278) ccw construction
  line L180 (-23.7959, 31.7391) -> (-25.6482, 32.1619) construction
  line L181 (-25.6482, 32.1619) -> (-24.7864, 35.9377) construction
  line L182 (-24.7864, 35.9377) -> (-22.934, 35.5149) construction
  arc A302 (-22.934, 35.5149) -> (-22.6762, 34.9595) centre (-22.4466, 35.4037) ccw construction
  arc A303 (-21.8674, 33.7126) -> (-22.6762, 34.9595) centre (-23.365, 33.627) ccw construction
  arc A304 (-21.8674, 33.7126) -> (-22.0528, 32.9001) centre (-21.2565, 33.1458) ccw construction
  arc A305 (-23.68, 27.5487) -> (-22.5687, 28.5356) centre (-23.9895, 29.0165) ccw construction
  arc A306 (-23.68, 27.5487) -> (-24.0764, 27.0819) centre (-23.5769, 27.0595) ccw construction
  line L183 (-24.0764, 27.0819) -> (-25.9745, 27.1672) construction
  line L184 (-25.9745, 27.1672) -> (-25.8007, 31.0362) construction
  line L185 (-25.8007, 31.0362) -> (-23.9026, 30.951) construction
  arc A307 (-23.9026, 30.951) -> (-23.5497, 30.4505) centre (-23.4031, 30.9286) ccw construction
  arc A308 (-22.5313, 29.3681) -> (-23.5497, 30.4505) centre (-23.9895, 29.0165) ccw construction
  arc A309 (-22.5313, 29.3681) -> (-22.5687, 28.5356) centre (-21.829, 28.9194) ccw construction
  arc A310 (-23.2142, 22.9796) -> (-22.2969, 24.149) centre (-23.7808, 24.3685) ccw construction
  arc A311 (-23.2142, 22.9796) -> (-23.5208, 22.4495) centre (-23.0253, 22.5166) ccw construction
  line L186 (-23.5208, 22.4495) -> (-25.4036, 22.1945) construction
  line L187 (-25.4036, 22.1945) -> (-25.9235, 26.0324) construction
  line L188 (-25.9235, 26.0324) -> (-24.0407, 26.2874) construction
  arc A312 (-24.0407, 26.2874) -> (-23.6041, 25.858) centre (-23.5452, 26.3546) ccw construction
  arc A313 (-22.4088, 24.9748) -> (-23.6041, 25.858) centre (-23.7808, 24.3685) ccw construction
  arc A314 (-22.4088, 24.9748) -> (-22.2969, 24.149) centre (-21.6377, 24.6588) ccw construction
  arc A315 (-21.94, 18.5671) -> (-21.2462, 19.8815) centre (-22.7454, 19.8325) ccw construction
  arc A316 (-21.94, 18.5671) -> (-22.147, 17.9908) centre (-21.6715, 18.1453) ccw construction
  line L189 (-22.147, 17.9908) -> (-23.954, 17.4036) construction
  line L190 (-23.954, 17.4036) -> (-25.1509, 21.0871) construction
  line L191 (-25.1509, 21.0871) -> (-23.3438, 21.6742) construction
  arc A317 (-23.3438, 21.6742) -> (-22.8376, 21.3296) centre (-22.8683, 21.8287) ccw construction
  arc A318 (-21.5038, 20.674) -> (-22.8376, 21.3296) centre (-22.7454, 19.8325) ccw construction
  arc A319 (-21.5038, 20.674) -> (-21.2462, 19.8815) centre (-20.6886, 20.5008) ccw construction
  arc A320 (-19.8984, 14.453) -> (-19.4505, 15.8701) centre (-20.9168, 15.5542) ccw construction
  arc A321 (-19.8984, 14.453) -> (-19.9992, 13.849) centre (-19.5589, 14.0859) ccw construction
  line L192 (-19.9992, 13.849) -> (-21.6723, 12.9486) construction
  line L193 (-21.6723, 12.9486) -> (-23.5076, 16.3591) construction
  line L194 (-23.5076, 16.3591) -> (-21.8345, 17.2595) construction
  arc A322 (-21.8345, 17.2595) -> (-21.2748, 17.0109) centre (-21.3942, 17.4964) ccw construction
  arc A323 (-19.8454, 16.604) -> (-21.2748, 17.0109) centre (-20.9168, 15.5542) ccw construction
  arc A324 (-19.8454, 16.604) -> (-19.4505, 15.8701) centre (-19.0124, 16.579) ccw construction
  arc A325 (-17.155, 10.7695) -> (-16.9673, 12.2439) centre (-18.3537, 11.6712) ccw construction
  arc A326 (-17.155, 10.7695) -> (-17.1463, 10.1572) centre (-16.7554, 10.469) ccw construction
  line L195 (-17.1463, 10.1572) -> (-18.6318, 8.9726) construction
  line L196 (-18.6318, 8.9726) -> (-21.0466, 12.0006) construction
  line L197 (-21.0466, 12.0006) -> (-19.5611, 13.1852) construction
  arc A327 (-19.5611, 13.1852) -> (-18.966, 13.0406) centre (-19.1702, 13.497) ccw construction
  arc A328 (-17.4869, 12.8954) -> (-18.966, 13.0406) centre (-18.3537, 11.6712) ccw construction
  arc A329 (-17.4869, 12.8954) -> (-16.9673, 12.2439) centre (-16.6629, 13.0196) ccw construction
  arc A330 (-13.7979, 7.6351) -> (-13.8766, 9.1193) centre (-15.1384, 8.3083) ccw construction
  arc A331 (-13.7979, 7.6351) -> (-13.6801, 7.0342) centre (-13.3511, 7.4108) ccw construction
  line L198 (-13.6801, 7.0342) -> (-14.9302, 5.6034) construction
  line L199 (-14.9302, 5.6034) -> (-17.8468, 8.1516) construction
  line L200 (-17.8468, 8.1516) -> (-16.5967, 9.5824) construction
  arc A332 (-16.5967, 9.5824) -> (-15.9854, 9.5463) centre (-16.2678, 9.9589) ccw construction
  arc A333 (-14.5041, 9.6676) -> (-15.9854, 9.5463) centre (-15.1384, 8.3083) ccw construction
  arc A334 (-14.5041, 9.6676) -> (-13.8766, 9.1193) centre (-13.7155, 9.937) ccw construction
  arc A335 (-9.9352, 5.1506) -> (-10.2776, 6.5968) centre (-11.3743, 5.5736) ccw construction
  arc A336 (-9.9352, 5.1506) -> (-9.712, 4.5803) centre (-9.4555, 5.0096) ccw construction
  line L201 (-9.712, 4.5803) -> (-10.6865, 2.9493) construction
  line L202 (-10.6865, 2.9493) -> (-14.0112, 4.9357) construction
  line L203 (-14.0112, 4.9357) -> (-13.0367, 6.5668) construction
  arc A337 (-13.0367, 6.5668) -> (-12.4288, 6.6404) centre (-12.7803, 6.996) ccw construction
  arc A338 (-10.9929, 7.0243) -> (-12.4288, 6.6404) centre (-11.3743, 5.5736) ccw construction
  arc A339 (-10.9929, 7.0243) -> (-10.2776, 6.5968) centre (-10.2651, 7.4301) ccw construction
  arc A340 (-5.6909, 3.3956) -> (-6.286, 4.7575) centre (-7.1824, 3.5548) ccw construction
  arc A341 (-5.6909, 3.3956) -> (-5.3694, 2.8744) centre (-5.1937, 3.3425) ccw construction
  line L204 (-5.3694, 2.8744) -> (-6.037, 1.0956) construction
  line L205 (-6.037, 1.0956) -> (-9.6631, 2.4564) construction
  line L206 (-9.6631, 2.4564) -> (-8.9954, 4.2353) construction
  arc A342 (-8.9954, 4.2353) -> (-8.4104, 4.4163) centre (-8.8198, 4.7034) ccw construction
  arc A343 (-7.0662, 5.0503) -> (-8.4104, 4.4163) centre (-7.1824, 3.5548) ccw construction
  arc A344 (-7.0662, 5.0503) -> (-6.286, 4.7575) centre (-6.4225, 5.5796) ccw construction
  arc A345 (-1.2015, 2.4267) -> (-2.0302, 3.6605) centre (-2.6974, 2.3171) ccw construction
  arc A346 (-1.2015, 2.4267) -> (-0.7921, 1.9713) centre (-0.7028, 2.4633) ccw construction
  line L207 (-0.7921, 1.9713) -> (-1.1313, 0.1018) construction
  line L208 (-1.1313, 0.1018) -> (-4.9421, 0.7934) construction
  line L209 (-4.9421, 0.7934) -> (-4.6028, 2.6628) construction
  arc A347 (-4.6028, 2.6628) -> (-4.0595, 2.9454) centre (-4.5135, 3.1548) ccw construction
  arc A348 (-2.8501, 3.8093) -> (-4.0595, 2.9454) centre (-2.6974, 2.3171) ccw construction
  arc A349 (-2.8501, 3.8093) -> (-2.0302, 3.6605) centre (-2.3113, 4.445) ccw construction
  circle A350 centre (1.9365, 27.8521) radius 27.8521
  circle A351 centre (1.9365, 27.8521) radius 26.0243